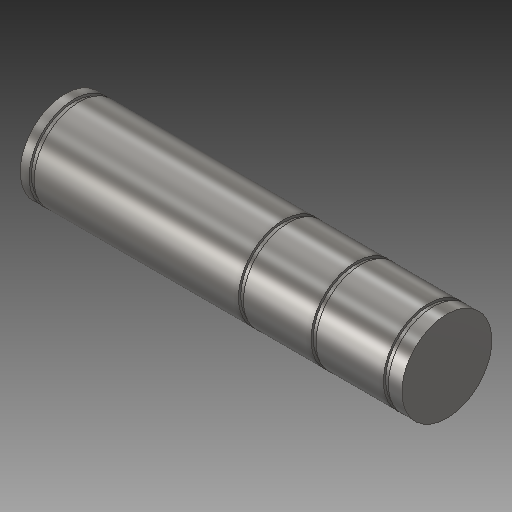
# Autodesk Inventor part: Center Axle
Saved by Autodesk Inventor 2019.4 (Build 234330000, 330)
## iProperties
Created: 2019-12-14
Part Number: Center Axle
Material: Steel, Mild
Document SubType Name: Modeling
Designer: admin
Density: 7.85 g/cm^3
Appearance: Semi-Polished
Author: admin
Autodesk Inventor part; units mm, degrees
ref_plane "YZ Plane" through (0, 0, 0) normal (1, 0, 0) x (0, 1, 0)
ref_plane "XZ Plane" through (0, 0, 0) normal (0, 1, 0) x (-1, 0, 0)
ref_plane "XY Plane" through (0, 0, 0) normal (0, 0, 1) x (1, 0, 0)
sketch "Sketch1" plane through (0, 0, 0) normal (0, 0, 1) x (1, 0, 0)
  line L0 (64.6, 10) -> (64.6, 9.5)
  line L1 (64.6, 9.5) -> (65.7, 9.5)
  line L2 (65.7, 9.5) -> (65.7, 10)
  line L3 (65.7, 10) -> (80.7, 10)
  line L4 (80.7, 10) -> (80.7, 9.5)
  line L5 (80.7, 9.5) -> (81.8, 9.5)
  line L6 (81.8, 9.5) -> (81.8, 10)
  line L7 (81.8, 10) -> (84.8, 10)
  line L8 (84.8, 10) -> (84.8, 0)
  line L9 (84.8, 0) -> (0, 0)
  line L10 (0, 10) -> (0, 0)
  line L11 (64.6, 10) -> (49.6, 10)
  line L12 (49.6, 10) -> (49.6, 9.5)
  line L13 (49.6, 9.5) -> (48.5, 9.5)
  line L14 (48.5, 9.5) -> (48.5, 10)
  line L15 (0, 10) -> (2, 10)
  line L16 (2, 10) -> (2, 9.5)
  line L17 (2, 9.5) -> (3.1, 9.5)
  line L18 (3.1, 9.5) -> (3.1, 10)
  line L19 (3.1, 10) -> (48.5, 10)
  dimension "d3" = 1.1
  dimension "d5" = 1.1
  dimension "d6" = 10
  dimension "d12" = 3
  dimension "d20" = 0.5
  dimension "d21" = 0.5
  dimension "d22" = 0.5
  dimension "d23" = 15
  dimension "d32" = 64.6
  dimension "d33" = 15
  dimension "d34" = 1.1
  dimension "d35" = 0.5
  dimension "d36" = 1.1
  dimension "d37" = 0.5
  dimension "d38" = 2
  constraints: 40 end point, 13 perpendicular, 6 point on line, 3 horizontal, 1 vertical
  measures "d3" distance of L0.end L1.end
  measures "d5" distance of L4.end L5.end
  measures "d6" distance between parallel lines of L9 L3
  measures "d12" distance of L6.end L7.end
  measures "d20" distance of L0.start L0.end
  measures "d21" distance of L3.end L4.end
  measures "d22" distance of L1.end L2.end
  measures "d23" distance of L2.end L3.end
  measures "d32" distance of L10.start L0.start
  measures "d33" distance of L0.start L11.end
  measures "d34" distance of L12.end L13.end
  measures "d35" distance of L11.end L12.end
  measures "d36" distance of L16.end L17.end
  measures "d37" distance of L15.end L16.end
  measures "d38" distance of L10.start L15.end
revolve "Revolution1" add sketch "Sketch1" angle 360 about axis through (84.8, 0, 0) along (-1, 0, 0)
body "Solid1"
